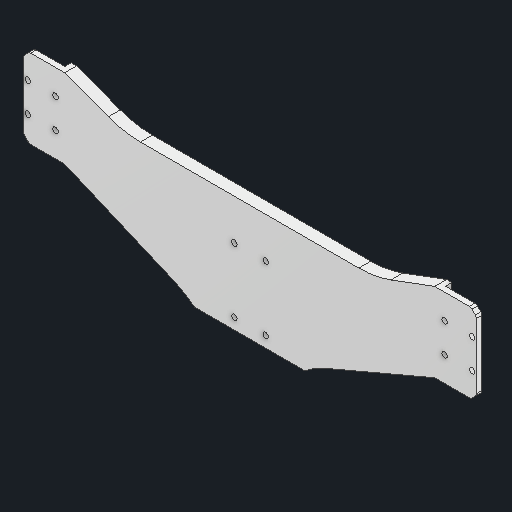
# Autodesk Inventor part: ZBridgePlate
Saved by Autodesk Inventor 2026.2 (Build 302298000, 298)
## iProperties
Created: 2026-03-10
Part Number: ZBridgePlate
Material: ABS Plastic
Document SubType Name: Modeling
Designer: gaoet
Density: 1.06 g/cm^3
Appearance: Smooth - White
Author: gaoet
Autodesk Inventor part; units mm, degrees
ref_plane "YZ Plane" through (0, 0, 0) normal (1, 0, 0) x (0, 1, 0)
ref_plane "XZ Plane" through (0, 0, 0) normal (0, 1, 0) x (-1, 0, 0)
ref_plane "XY Plane" through (0, 0, 0) normal (0, 0, 1) x (1, 0, 0)
sketch "Sketch1" plane through (0, 0, 0) normal (0, 0, 1) x (1, 0, 0)
  line L0 (-123, 21.5) -> (123, 21.5)
  line L1 (123, 21.5) -> (123, -21.5)
  line L2 (123, -21.5) -> (-123, -21.5)
  line L3 (-123, -21.5) -> (-123, 21.5)
  line L4 (-123, 21.5) -> (123, -21.5) construction
  line L5 (123, 21.5) -> (-123, -21.5) construction
  line L6 (0, -155.5635) -> (155.5635, 0) construction
  line L7 (155.5635, 0) -> (0, 155.5635) construction
  line L8 (0, 155.5635) -> (-155.5635, 0) construction
  line L9 (-155.5635, 0) -> (0, -155.5635) construction
  line L10 (0, -155.5635) -> (0, 155.5635) construction
  line L11 (155.5635, 0) -> (-155.5635, 0) construction
  line L12 (0, -155.5635) -> (220, -155.5635) construction
  line L13 (-120.75, -8) -> (120.75, -8)
  line L14 (120.75, -8) -> (120.75, 8)
  line L15 (120.75, 8) -> (-120.75, 8)
  line L16 (-120.75, 8) -> (-120.75, -8)
  line L17 (-120.75, -8) -> (120.75, 8) construction
  line L18 (120.75, -8) -> (-120.75, 8) construction
  line L19 (-105.75, -8) -> (105.75, -8)
  line L20 (105.75, -8) -> (105.75, 8)
  line L21 (105.75, 8) -> (-105.75, 8)
  line L22 (-105.75, 8) -> (-105.75, -8)
  line L23 (-105.75, -8) -> (105.75, 8) construction
  line L24 (105.75, -8) -> (-105.75, 8) construction
  line L25 (-100.75, 21.5) -> (-100.75, -21.5)
  line L26 (100.3399, 21.5) -> (100.3399, -21.5)
  line L27 (-100.75, 21.5) -> (-20.205, -8.5)
  line L28 (-20.205, -8.5) -> (19.795, -8.5)
  line L29 (19.795, -8.5) -> (100.3399, 21.5)
  line L30 (-100.75, -21.5) -> (-30.205, -51.5)
  line L31 (-30.205, -51.5) -> (29.795, -51.5)
  line L32 (29.795, -51.5) -> (100.3399, -21.5)
  point P0 (0, 0)
  point P1 (64.0947, 8)
  point P2 (-64.5048, 8)
  dimension "d0" = 246
  dimension "d1" = 220
  dimension "d2" = 45
  dimension "d3" = 220
  dimension "d4" = 43
  dimension "d5" = 241.5
  dimension "d6" = 16
  dimension "d7" = 15
  dimension "d29" = 2.25
  dimension "d30" = 5
  dimension "d31" = 5.4101
  dimension "d32" = 30
  dimension "d33" = 30
  dimension "d34" = 40
  dimension "d35" = 60
  constraints: 66 end point, 8 midpoint, 8 parallel, 6 horizontal, 5 perpendicular, 5 point on line, 3 equal length, 1 vertical
  measures "d0" distance of L1.end L2.end
  measures "d1" distance of L6.start L6.end
  measures "d2" angle of L12 L6
  measures "d3" distance of L7.end L6.end
  measures "d4" distance of L2.end L0.start
  measures "d5" distance of L15.end L14.end
  measures "d6" distance of L14.end L13.end
  measures "d7" distance between parallel lines of L14 L20
  measures "d29" distance between parallel lines of L3 L16
  measures "d30" distance between parallel lines of L22 L25
  measures "d31" distance between parallel lines of L26 L20
  measures "d32" distance between parallel lines of L0 L28
  measures "d33" distance between parallel lines of L31 L2
  measures "d34" distance of L27.end L28.end
  measures "d35" distance of L30.end L31.end
extrude "Extrusion1" add sketch "Sketch1" along normal blind 6.5 contours L0 L25 L15 L16 L13 L2 L3 | L27 L15 L25 | L0 L1 L2 L26 L13 L14 L15 | L26 L15 L29 | L25 L13 L22 L15 | L15 L27 L13 L25 | L25 L13 L27 L28 L29 L26 L2 | L2 L32 L31 L30 | L26 L13 L29 L15 | L15 L20 L13 L26 | L22 L13 L16 L15 | L15 L14 L13 L20
hole "Hole1" at (-105.75, -8, 0) at (-120.75, -8, 0) at (-120.75, 8, 0) at (-105.75, 8, 0) at (120.75, -8, 0) at (105.75, -8, 0) at (105.75, 8, 0) at (120.75, 8, 0) direction (0, 0, 1) diameter 3 end through all
sketch "Sketch2" plane through (0, 0, 6.5) normal (0, 0, 1) x (1, 0, 0)
  line L0 (123, 21.5) -> (-123, 21.5) projected
  line L1 (-12.5, -21.5) -> (12.5, -21.5)
  line L2 (12.5, -21.5) -> (12.5, 21.5)
  line L3 (12.5, 21.5) -> (-12.5, 21.5)
  line L4 (-12.5, 21.5) -> (-12.5, -21.5)
  line L5 (-12.5, -21.5) -> (12.5, 21.5) construction
  line L6 (12.5, -21.5) -> (-12.5, 21.5) construction
  line L7 (12.5, -21.5) -> (12.5, -51.5)
  line L8 (-12.5, -21.5) -> (-12.5, -51.5)
  circle A0 centre (120.75, 8) radius 1.5 projected
  circle A1 centre (105.75, 8) radius 1.5 projected
  circle A2 centre (105.75, -8) radius 1.5 projected
  circle A3 centre (120.75, -8) radius 1.5 projected
  circle A4 centre (-105.75, 8) radius 1.5 projected
  circle A5 centre (-120.75, 8) radius 1.5 projected
  circle A6 centre (-120.75, -8) radius 1.5 projected
  circle A7 centre (-105.75, -8) radius 1.5 projected
  line L9 (-20.205, -8.5) -> (-100.75, 21.5) projected
  line L10 (-100.75, 21.5) -> (-123, 21.5) projected
  line L11 (-123, 21.5) -> (-123, -21.5) projected
  line L12 (-123, -21.5) -> (-100.75, -21.5) projected
  line L13 (-100.75, -21.5) -> (-30.205, -51.5) projected
  line L14 (-30.205, -51.5) -> (29.795, -51.5) projected
  line L15 (29.795, -51.5) -> (100.3399, -21.5) projected
  line L16 (100.3399, -21.5) -> (123, -21.5) projected
  line L17 (123, -21.5) -> (123, 21.5) projected
  line L18 (123, 21.5) -> (100.3399, 21.5) projected
  line L19 (100.3399, 21.5) -> (19.795, -8.5) projected
  line L20 (19.795, -8.5) -> (-20.205, -8.5) projected
  point P0 (0, 0)
  dimension "d17" = 25
  constraints: 16 end point, 3 point on line, 2 midpoint, 2 parallel, 2 perpendicular, 2 vertical, 1 horizontal
  measures "d17" distance of L3.end L2.end
sketch "Sketch4" plane through (0, 0, 0) normal (0, 0, -1) x (-1, 0, 0)
  circle A0 centre (-120.75, 8) radius 1.5 projected
  circle A1 centre (-105.75, 8) radius 1.5 projected
  circle A2 centre (-105.75, -8) radius 1.5 projected
  circle A3 centre (-120.75, -8) radius 1.5 projected
  circle A4 centre (105.75, 8) radius 1.5 projected
  circle A5 centre (120.75, 8) radius 1.5 projected
  circle A6 centre (120.75, -8) radius 1.5 projected
  circle A7 centre (105.75, -8) radius 1.5 projected
  line L0 (-19.795, -8.5) -> (20.205, -8.5) projected
  line L1 (-100.3399, 21.5) -> (-19.795, -8.5) projected
  line L2 (-123, 21.5) -> (-100.3399, 21.5) projected
  line L3 (-123, -21.5) -> (-123, 21.5) projected
  line L4 (-100.3399, -21.5) -> (-123, -21.5) projected
  line L5 (-29.795, -51.5) -> (-100.3399, -21.5) projected
  line L6 (30.205, -51.5) -> (-29.795, -51.5) projected
  line L7 (100.75, -21.5) -> (30.205, -51.5) projected
  line L8 (123, -21.5) -> (100.75, -21.5) projected
  line L9 (123, 21.5) -> (123, -21.5) projected
  line L10 (100.75, 21.5) -> (123, 21.5) projected
  line L11 (20.205, -8.5) -> (100.75, 21.5) projected
  line L12 (12.5, 21.5) -> (12.5, -21.5) projected
  line L13 (-12.5, -21.5) -> (-12.5, 21.5) projected
  line L14 (-12.5, -21.5) -> (-12.5, -51.5) projected
  line L15 (12.5, -21.5) -> (12.5, -51.5) projected
  point P0 (0, 0)
  point P1 (12.5, -8.5)
  point P2 (-12.5, -8.5)
extrude "Extrusion3" cut sketch "Sketch4" against normal blind 2.5 contours L0 L12 L15 L6 L14 L13
sketch "Sketch5" plane through (0, 0, 2.5) normal (0, 0, -1) x (-1, 0, 0)
  line L0 (12.5, -8.5) -> (12.5, -51.5) projected
  line L1 (-12.5, -8.5) -> (12.5, -8.5) projected
  line L2 (-12.5, -51.5) -> (-12.5, -8.5) projected
  line L3 (12.5, -51.5) -> (-12.5, -51.5) projected
  line L4 (8.5, -12.5) -> (-8.5, -12.5)
  line L5 (-8.5, -12.5) -> (-8.5, -47.5)
  line L6 (-8.5, -47.5) -> (8.5, -47.5)
  line L7 (8.5, -47.5) -> (8.5, -12.5)
  line L8 (8.5, -12.5) -> (-8.5, -47.5) construction
  line L9 (-8.5, -12.5) -> (8.5, -47.5) construction
  point P0 (0, 0)
  point P1 (0, -30)
  dimension "d43" = 4
  dimension "d44" = 4
  dimension "d45" = 4
  constraints: 12 end point, 2 midpoint, 2 parallel, 1 horizontal, 1 perpendicular, 1 vertical alignment
  measures "d43" distance between parallel lines of L3 L6
  measures "d44" distance between parallel lines of L2 L5
  measures "d45" distance between parallel lines of L1 L4
hole "Hole3" at (-8.5, -47.5, 2.5) at (8.5, -47.5, 2.5) at (8.5, -12.5, 2.5) at (-8.5, -12.5, 2.5) direction (0, 0, 1) diameter 3 end through all
sketch "Sketch6" plane through (0, 0, 0) normal (0, 0, -1) x (-1, 0, 0)
  line L0 (-12.5, -51.5) -> (-12.5, -8.5) projected
  line L1 (-19.795, -8.5) -> (-12.5, -8.5) projected
  line L2 (-100.3399, 21.5) -> (-19.795, -8.5) projected
  line L3 (-123, 21.5) -> (-100.3399, 21.5) projected
  line L4 (-123, -21.5) -> (-123, 21.5) projected
  line L5 (-100.3399, -21.5) -> (-123, -21.5) projected
  line L6 (-29.795, -51.5) -> (-100.3399, -21.5) projected
  line L7 (-12.5, -51.5) -> (-29.795, -51.5) projected
  circle A0 centre (-120.75, 8) radius 1.5 projected
  circle A1 centre (-105.75, 8) radius 1.5 projected
  circle A2 centre (-105.75, -8) radius 1.5 projected
  circle A3 centre (-120.75, -8) radius 1.5 projected
  line L8 (12.5, -8.5) -> (12.5, -51.5) projected
  line L9 (30.205, -51.5) -> (12.5, -51.5) projected
  line L10 (100.75, -21.5) -> (30.205, -51.5) projected
  line L11 (123, -21.5) -> (100.75, -21.5) projected
  line L12 (123, 21.5) -> (123, -21.5) projected
  line L13 (100.75, 21.5) -> (123, 21.5) projected
  line L14 (20.205, -8.5) -> (100.75, 21.5) projected
  line L15 (12.5, -8.5) -> (20.205, -8.5) projected
  circle A4 centre (105.75, -8) radius 1.5 projected
  circle A5 centre (120.75, -8) radius 1.5 projected
  circle A6 centre (120.75, 8) radius 1.5 projected
  circle A7 centre (105.75, 8) radius 1.5 projected
  line L16 (-100.3399, -21.5) -> (-100.3399, 21.5)
  line L17 (100.75, -21.5) -> (100.75, 21.5)
  line L18 (123, -21.5) -> (100.75, -21.5) projected
  line L19 (103.6601, 21.5) -> (103.6601, -21.5)
  line L20 (-103.25, 21.5) -> (-103.25, -21.5)
  point P0 (0, 0)
  dimension "d55" = 2.9101
  dimension "d56" = 2.9101
  constraints: 8 end point, 4 point on line, 2 perpendicular, 2 vertical
  measures "d55" distance between parallel lines of L16 L20
  measures "d56" distance between parallel lines of L17 L19
extrude "Extrusion4" cut sketch "Sketch6" against normal blind 3.5 contours L5 L4 L3 L20 | L13 L12 L11 L19
sketch "Sketch7" plane through (-30.205, -51.5, 6.5) normal (0, -1, 0) x (1, 0, 0)
  line L0 (17.705, -6.5) -> (17.705, -4) projected
  line L1 (17.705, -4) -> (42.705, -4) projected
  line L2 (42.705, -4) -> (42.705, -6.5) projected
  line L3 (42.705, -6.5) -> (60, -6.5) projected
  line L4 (60, -6.5) -> (60, 0) projected
  line L5 (0, 0) -> (60, 0) projected
  line L6 (0, -6.5) -> (0, 0) projected
  line L7 (0, -6.5) -> (17.705, -6.5) projected
  point P0 (30.205, -6.5)
extrude "Extrusion5" add sketch "Sketch7" along normal blind 2
chamfer "Chamfer1" distance 2 angle 45 2 edges at (-30.205, -51.5, 3.25) (29.795, -51.5, 3.25)
sketch "Sketch8" plane through (0, 0, 2.5) normal (0, 0, -1) x (-1, 0, 0)
  line L0 (0, 160.3722) -> (-155.5635, 4.8087)
  line L1 (-155.5635, 4.8087) -> (0, -150.7548)
  line L2 (0, -150.7548) -> (155.5635, 4.8087)
  line L3 (155.5635, 4.8087) -> (0, 160.3722)
  line L4 (0, 160.3722) -> (0, -150.7548) construction
  line L5 (-155.5635, 4.8087) -> (155.5635, 4.8087) construction
  point P0 (0, 0)
  point P1 (0, 4.8087)
  dimension "d62" = 220
  constraints: 12 end point, 2 midpoint, 2 parallel, 1 horizontal, 1 perpendicular, 1 vertical
  measures "d62" distance of L0.end L1.end
fillet "Fillet2" radius 50 4 edges at (-20.205, -8.5, 3.25) (19.795, -8.5, 3.25) (-32.0454, -50.7174, 3.25) (31.6354, -50.7174, 3.25)
sketch "Sketch9" plane through (0, 0, 6.5) normal (0, 0, 1) x (1, 0, 0)
  circle A0 centre (-8.5, -12.5) radius 1.5 projected
  circle A1 centre (8.5, -12.5) radius 1.5 projected
  circle A2 centre (8.5, -47.5) radius 1.5 projected
  circle A3 centre (-8.5, -47.5) radius 1.5 projected
  circle A4 centre (120.75, 8) radius 1.5 projected
  circle A5 centre (105.75, 8) radius 1.5 projected
  circle A6 centre (105.75, -8) radius 1.5 projected
  circle A7 centre (120.75, -8) radius 1.5 projected
  circle A8 centre (-105.75, 8) radius 1.5 projected
  circle A9 centre (-120.75, 8) radius 1.5 projected
  circle A10 centre (-120.75, -8) radius 1.5 projected
  circle A11 centre (-105.75, -8) radius 1.5 projected
  line L0 (10.7857, -8.5) -> (-11.1958, -8.5) projected
  arc A12 (-28.6477, -5.3554) -> (-11.1958, -8.5) centre (-11.1958, 41.5) ccw projected
  line L1 (-28.6477, -5.3554) -> (-100.75, 21.5) projected
  line L2 (-100.75, 21.5) -> (-123, 21.5) projected
  line L3 (-123, 21.5) -> (-123, -21.5) projected
  line L4 (-123, -21.5) -> (-100.75, -21.5) projected
  line L5 (-100.75, -21.5) -> (-41.8538, -46.5462) projected
  arc A13 (-30.205, -53.5) -> (-41.8538, -46.5462) centre (-61.421, -92.5585) ccw projected
  line L6 (29.795, -53.5) -> (-30.205, -53.5) projected
  arc A14 (41.4437, -46.5462) -> (29.795, -53.5) centre (61.0109, -92.5585) ccw projected
  line L7 (41.4437, -46.5462) -> (100.3399, -21.5) projected
  line L8 (100.3399, -21.5) -> (123, -21.5) projected
  line L9 (123, -21.5) -> (123, 21.5) projected
  line L10 (123, 21.5) -> (100.3399, 21.5) projected
  line L11 (100.3399, 21.5) -> (28.2376, -5.3554) projected
  arc A15 (10.7857, -8.5) -> (28.2376, -5.3554) centre (10.7857, 41.5) ccw projected
  point P0 (0, 0)
sketch "Sketch10" plane through (0, 0, 6.5) normal (0, 0, 1) x (1, 0, 0)
  circle A0 centre (-8.5, -12.5) radius 1.5 projected
  circle A1 centre (8.5, -12.5) radius 1.5 projected
  circle A2 centre (8.5, -47.5) radius 1.5 projected
  circle A3 centre (-8.5, -47.5) radius 1.5 projected
  circle A4 centre (120.75, 8) radius 1.5 projected
  circle A5 centre (105.75, 8) radius 1.5 projected
  circle A6 centre (105.75, -8) radius 1.5 projected
  circle A7 centre (120.75, -8) radius 1.5 projected
  circle A8 centre (-105.75, 8) radius 1.5 projected
  circle A9 centre (-120.75, 8) radius 1.5 projected
  circle A10 centre (-120.75, -8) radius 1.5 projected
  circle A11 centre (-105.75, -8) radius 1.5 projected
  line L0 (10.7857, -8.5) -> (-11.1958, -8.5) projected
  arc A12 (-28.6477, -5.3554) -> (-11.1958, -8.5) centre (-11.1958, 41.5) ccw projected
  line L1 (-28.6477, -5.3554) -> (-100.75, 21.5) projected
  line L2 (-100.75, 21.5) -> (-123, 21.5) projected
  line L3 (-123, 21.5) -> (-123, -21.5) projected
  line L4 (-123, -21.5) -> (-100.75, -21.5) projected
  line L5 (-100.75, -21.5) -> (-41.8538, -46.5462) projected
  arc A13 (-30.205, -53.5) -> (-41.8538, -46.5462) centre (-61.421, -92.5585) ccw projected
  line L6 (29.795, -53.5) -> (-30.205, -53.5) projected
  arc A14 (41.4437, -46.5462) -> (29.795, -53.5) centre (61.0109, -92.5585) ccw projected
  line L7 (41.4437, -46.5462) -> (100.3399, -21.5) projected
  line L8 (100.3399, -21.5) -> (123, -21.5) projected
  line L9 (123, -21.5) -> (123, 21.5) projected
  line L10 (123, 21.5) -> (100.3399, 21.5) projected
  line L11 (100.3399, 21.5) -> (28.2376, -5.3554) projected
  arc A15 (10.7857, -8.5) -> (28.2376, -5.3554) centre (10.7857, 41.5) ccw projected
  line L12 (-68.532, 9.5) -> (68.1219, 9.5)
  point P0 (0, 0)
  dimension "d64" = 18
  constraints: 2 end point, 2 point on line, 1 horizontal
  measures "d64" distance between parallel lines of L0 L12
extrude "Extrusion6" add sketch "Sketch10" against normal up to surface (6.5 mm away) contours L0 A12 L1 L12 L11 A15
fillet "Fillet3" radius 50 2 edges at (-68.532, 9.5, 3.25) (68.1219, 9.5, 3.25)
chamfer "Chamfer2" distance 3 angle 45 4 edges at (123, -21.5, 5) (123, 21.5, 5) (-123, -21.5, 5) (-123, 21.5, 5)
fillet "Fillet4" radius 2 8 edges at (-120, -21.5, 5) (-123, -18.5, 5) (-123, 18.5, 5) (-120, 21.5, 5) (120, 21.5, 5) (123, 18.5, 5) (120, -21.5, 5) (123, -18.5, 5)
equation "\"d33\" = d32"
equation "\"d44\" = d43"
equation "\"d45\" = d44"
body "Solid1"
